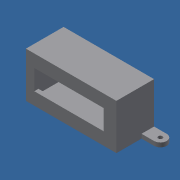
# Autodesk Inventor part: PSUBracket
Saved by Autodesk Inventor 2021 (Build 250183000, 183)
## iProperties
Created: 2022-09-10
Part Number: PSUBracket
Material: Generic
Document SubType Name: Modeling
Designer: Nathann
Density: 1 g/cm^3
Appearance: Default
Author: Nathann
Autodesk Inventor part; units mm, degrees
ref_plane "YZ Plane" through (0, 0, 0) normal (1, 0, 0) x (0, 1, 0)
ref_plane "XZ Plane" through (0, 0, 0) normal (0, 1, 0) x (-1, 0, 0)
ref_plane "XY Plane" through (0, 0, 0) normal (0, 0, 1) x (1, 0, 0)
sketch "Sketch1" plane through (0, 0, 0) normal (0, 0, 1) x (1, 0, 0)
  line L0 (0, 0) -> (-98, 0)
  line L1 (-98, 0) -> (-98, 44)
  line L2 (-98, 44) -> (0, 44)
  line L3 (0, 44) -> (0, 0)
  line L4 (5, -5) -> (-103, -5)
  line L5 (-103, -5) -> (-103, 49)
  line L6 (-103, 49) -> (5, 49)
  line L7 (5, 49) -> (5, -5)
  dimension "d0" = 98
  dimension "d1" = 44
  dimension "d2" = 5
  dimension "d3" = 5
  dimension "d4" = 5
  dimension "d5" = 5
  constraints: 16 end point, 4 parallel, 2 horizontal, 2 perpendicular
  measures "d0" distance of L1.end L2.end
  measures "d1" distance of L0.end L1.end
  measures "d2" distance between parallel lines of L4 L0
  measures "d3" distance between parallel lines of L7 L3
  measures "d4" distance between parallel lines of L2 L6
  measures "d5" distance between parallel lines of L5 L1
extrude "Extrusion1" add sketch "Sketch1" along normal blind 40
sketch "Sketch2" plane through (0, 0, 40) normal (0, 0, 1) x (1, 0, 0)
  line L0 (5, 49) -> (-103, 49) projected
  line L1 (5, -5) -> (-103, -5)
  line L2 (-103, -5) -> (-103, 49)
  line L3 (-103, 49) -> (5, 49)
  line L4 (5, 49) -> (5, -5)
  line L5 (-93, 34) -> (-10, 34)
  line L6 (-10, 34) -> (-10, 10)
  line L7 (-10, 10) -> (-93, 10)
  line L8 (-93, 10) -> (-93, 34)
  point P0 (0, 0)
  dimension "d10" = 10
  dimension "d11" = 15
  dimension "d12" = 15
  dimension "d13" = 15
  constraints: 16 end point, 4 parallel, 2 horizontal, 2 perpendicular
  measures "d10" distance between parallel lines of L2 L8
  measures "d11" distance between parallel lines of L4 L6
  measures "d12" distance between parallel lines of L0 L5
  measures "d13" distance between parallel lines of L1 L7
extrude "Extrusion2" add sketch "Sketch2" along normal blind 5
sketch "Sketch3" plane through (-103, -5, 0) normal (0, -1, 0) x (1, 0, 0)
  line L0 (108, 0) -> (108, 45) projected
  line L1 (108, 0) -> (123, 0)
  line L2 (123, 0) -> (123, 15)
  line L3 (123, 15) -> (108, 15)
  line L4 (108, 15) -> (108, 0)
  circle A0 centre (123, 7.5) radius 7.5
  circle A1 centre (123, 7.5) radius 2.5
  line L5 (108, 45) -> (0, 45) projected
  line L6 (54, 45) -> (54, 61.5977)
  line L7 (0, 0) -> (-15, 0)
  line L8 (-15, 0) -> (-15, 15)
  line L9 (-15, 15) -> (0, 15)
  line L10 (0, 15) -> (0, 0)
  circle A2 centre (-15, 7.5) radius 7.5
  circle A3 centre (-15, 7.5) radius 2.5
  point P0 (103, 0)
  point P1 (5, 0)
  dimension "d14" = 15
  dimension "d15" = 15
  dimension "d16" = 5
  constraints: 18 end point, 7 symmetric about line, 2 centre point, 2 coincident, 2 midpoint, 2 parallel, 2 vertical, 1 horizontal, 1 perpendicular, 7 other
  measures "d14" distance between parallel lines of L3 L1
  measures "d15" distance between parallel lines of L0 L2
  measures "d16" diameter of A1
extrude "Extrusion3" add sketch "Sketch3" against normal blind 5 contours L0 L3 A0 L1 | A0 L2 A1 | L2 A1 A0 | L7 A2 L9 L10 | A2 L8 A3 | L8 A3 A2
body "Solid1"
